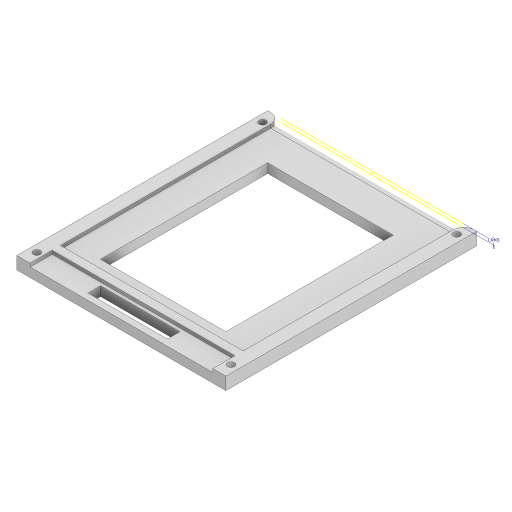
# Autodesk Inventor part: Scanner_Test_Bot
Saved by Autodesk Inventor 2023 (Build 270158000, 158)
## iProperties
Created: 2022-09-22
Part Number: Scanner_Test_Bot
Material: Generic
Document SubType Name: Modeling
Designer: Vking
Density: 1 g/cm^3
Appearance: Default
Author: Vking
Autodesk Inventor part; units mm, degrees
ref_plane "YZ Plane" through (0, 0, 0) normal (1, 0, 0) x (0, 1, 0)
ref_plane "XZ Plane" through (0, 0, 0) normal (0, 1, 0) x (-1, 0, 0)
ref_plane "XY Plane" through (0, 0, 0) normal (0, 0, 1) x (1, 0, 0)
sketch "Sketch1" plane through (0, 0, 0) normal (0, 0, 1) x (1, 0, 0)
  line L0 (-31.75, 5.08) -> (31.75, 5.08)
  line L1 (31.75, 5.08) -> (31.75, -5.08)
  line L2 (31.75, -5.08) -> (-31.75, -5.08)
  line L3 (-31.75, -5.08) -> (-31.75, 5.08)
  point P0 (0, 0)
  dimension "d0" = 63.5
  dimension "d3" = 31.75
  dimension "d4" = 10.16
  dimension "d17" = 5.08
  constraints: 8 end point, 2 parallel, 1 horizontal, 1 perpendicular
  measures "d0" distance of L0.start L0.end
  measures "d3" distance from line of L3 point (0, 0)
  measures "d4" distance of L0.end L1.end
  measures "d17" distance from line of point (0, 0) L2
extrude "Extrusion1" add sketch "Sketch1" along normal blind 76.2
sketch "Sketch3" plane through (0, 0, 76.2) normal (0, 0, 1) x (1, 0, 0)
  line L0 (-27.75, 0.3875) -> (27.75, 0.3875)
  line L1 (27.75, 0.3875) -> (27.75, -0.3745)
  line L2 (27.75, -0.3745) -> (-27.75, -0.3745)
  line L3 (-27.75, -0.3745) -> (-27.75, 0.3875)
  line L4 (-31.75, 5.08) -> (-31.75, -5.08) projected
  point P0 (0, 0)
  point P1 (-27.75, 0.0065)
  dimension "d6" = 0.762
  dimension "d7" = 55.5
  dimension "d8" = 4
  constraints: 8 end point, 2 parallel, 1 horizontal, 1 midpoint, 1 perpendicular
  measures "d6" distance between parallel lines of L2 L0
  measures "d7" distance of L0.start L0.end
  measures "d8" distance from line of L4 point (-27.75, 0.006)
extrude "Extrusion2" cut sketch "Sketch3" against normal blind 85.1
sketch "Sketch8" plane through (0, 0, 76.2) normal (0, 0, 1) x (1, 0, 0)
  line L0 (27.75, 0.3875) -> (27.75, -0.3745) projected
  line L1 (27.75, -0.3745) -> (-27.75, -0.3745) projected
  line L2 (-27.75, -0.3745) -> (-27.75, 0.3875) projected
  line L3 (-27.75, 0.3875) -> (27.75, 0.3875) projected
  line L4 (-31.75, -5.08) -> (31.75, -5.08) projected
  line L5 (31.75, -5.08) -> (31.75, 5.08) projected
  line L6 (31.75, 5.08) -> (-31.75, 5.08) projected
  line L7 (-31.75, 5.08) -> (-31.75, -5.08) projected
  line L8 (-31.75, 5.08) -> (31.75, 5.08)
  line L9 (31.75, 5.08) -> (31.75, 0.3875)
  line L10 (31.75, 0.3875) -> (-31.75, 0.3875)
  line L11 (-31.75, 0.3875) -> (-31.75, 5.08)
  point P0 (0, 0)
  point P1 (-31.75, 0.3875)
  dimension "d30" = 0
  constraints: 8 end point, 2 parallel, 1 horizontal, 1 perpendicular, 1 point on line
  measures "d30" distance between parallel lines of L3 L10
extrude "Extrusion6" cut sketch "Sketch8" against normal blind 76.2 contours L3 L10 L7 L6 L5
sketch "Sketch9" plane through (0, 0, 76.2) normal (0, 0, 1) x (1, 0, 0)
  line L0 (-31.75, 0.3875) -> (-31.75, -5.08) projected
  line L1 (31.75, -5.08) -> (31.75, 0.3875) projected
  line L2 (-31.75, -5.08) -> (31.75, -5.08)
  line L3 (31.75, -5.08) -> (31.75, -3.175)
  line L4 (31.75, -3.175) -> (-31.75, -3.175)
  line L5 (-31.75, -3.175) -> (-31.75, -5.08)
  point P0 (0, 0)
  dimension "d33" = 1.905
  constraints: 8 end point, 2 parallel, 1 horizontal, 1 perpendicular, 1 point on line
  measures "d33" distance between parallel lines of L2 L4
extrude "Extrusion7" cut sketch "Sketch9" against normal blind 76.2
sketch "Sketch10" plane through (-27.75, -0.3745, 76.2) normal (0, 1, 0) x (1, 0, 0)
  line L0 (59.5, 76.2) -> (-4, 76.2) projected
  line L1 (-4, 76.2) -> (59.5, 76.2)
  line L2 (59.5, 76.2) -> (59.5, 0)
  line L3 (59.5, 0) -> (-4, 0)
  line L4 (-4, 0) -> (-4, 76.2)
  line L5 (8.7, 12.7) -> (46.8, 12.7)
  line L6 (46.8, 12.7) -> (46.8, 63.5)
  line L7 (46.8, 63.5) -> (8.7, 63.5)
  line L8 (8.7, 63.5) -> (8.7, 12.7)
  dimension "d46" = 12.7
  constraints: 16 end point, 4 parallel, 2 perpendicular, 1 horizontal, 3 other
  measures "d46" distance between parallel lines of L3 L5
extrude "Extrusion8" cut sketch "Sketch10" against normal blind 25.4 contours L8 L7 L6 L5
fillet "Fillet3" radius 3.175 3 edges at (0, -0.3745, 0) (-27.75, 0.0065, 0) (27.75, 0.0065, 0)
sketch "Sketch11" plane through (-27.75, -0.3745, 76.2) normal (0, 1, 0) x (1, 0, 0)
  line L0 (15.6845, 1.905) -> (39.8145, 1.905)
  line L1 (39.8145, 1.905) -> (39.8145, 5.715)
  line L2 (39.8145, 5.715) -> (15.6845, 5.715)
  line L3 (15.6845, 5.715) -> (15.6845, 1.905)
  line L4 (55.5, 0) -> (0, 0) projected
  line L5 (0, 0) -> (0, 73.025) projected
  line L6 (-4, 0) -> (-4, 76.2) projected
  point P0 (27.75, 76.2)
  dimension "d47" = 1.905
  dimension "d48" = 3.81
  dimension "d51" = 24.13
  dimension "d52" = 15.6845
  dimension "d67" = 19.6845
  constraints: 8 end point, 2 parallel, 1 horizontal, 1 perpendicular
  measures "d47" distance between parallel lines of L4 L0
  measures "d48" distance between parallel lines of L0 L2
  measures "d51" distance of L1.end L2.end
  measures "d52" distance between parallel lines of L5 L3
  measures "d67" distance between parallel lines of L6 L3
extrude "Extrusion9" cut sketch "Sketch11" against normal blind 25.4
sketch "Sketch13" plane through (-31.75, -3.175, 76.2) normal (0, -1, 0) x (1, 0, 0)
  circle A0 centre (61.25, -3.81) radius 1.05
  line L0 (63.5, 0) -> (59, 0)
  circle A1 centre (2.25, -3.81) radius 1.05
  line L1 (4.5, 0) -> (0, 0)
  circle A2 centre (61.25, -72.39) radius 1.05
  line L2 (59, -76.2) -> (63.5, -76.2)
  line L3 (59, 0) -> (59, -76.2)
  circle A3 centre (2.25, -72.39) radius 1.05
  line L4 (0, 0) -> (0, -76.2)
  line L5 (0, -76.2) -> (4.5, -76.2)
  line L6 (50.8, -12.7) -> (50.8, -63.5)
  line L7 (50.8, -63.5) -> (12.7, -63.5)
  line L8 (12.7, -63.5) -> (12.7, -12.7)
  line L9 (12.7, -12.7) -> (50.8, -12.7)
  line L10 (63.5, 0) -> (0, 0)
  line L11 (0, 0) -> (0, -76.2)
  line L12 (63.5, -76.2) -> (0, -76.2)
  line L13 (63.5, 0) -> (63.5, -76.2)
  point P0 (31.75, -76.2)
  point P1 (31.75, -76.2)
  dimension "d53" = 2.1
  dimension "d54" = 3.81
  dimension "d55" = 2.25
  dimension "d56" = 2.25
  dimension "d57" = 2.1
  dimension "d58" = 3.81
  dimension "d59" = 2.1
  dimension "d60" = 2.1
  dimension "d61" = 3.81
  dimension "d62" = 3.81
  dimension "d63" = 2.25
  dimension "d64" = 2.25
  constraints: 28 end point, 4 centre point, 1 coincident
  measures "d53" diameter of A2
  measures "d54" distance from line of L2 A2.centre
  measures "d55" distance from line of A2.centre L3
  measures "d56" distance from line of L4 A3.centre
  measures "d57" diameter of A3
  measures "d58" distance from line of L5 A3.centre
  measures "d59" diameter of A1
  measures "d60" diameter of A0
  measures "d61" distance from line of A1.centre L1
  measures "d62" distance from line of A0.centre L0
  measures "d63" distance from line of L3 A0.centre
  measures "d64" distance from line of L4 A1.centre
extrude "Extrusion10" cut sketch "Sketch13" against normal blind 25.4 contours A0 | A1 | A2 | A3
sketch "Sketch14" plane through (-31.75, 0.3875, 76.2) normal (0, 1, 0) x (1, 0, 0)
  circle A0 centre (2.25, 3.81) radius 1.05 projected
  circle A1 centre (2.25, 72.39) radius 1.05 projected
  arc A2 (4, 73.025) -> (0.825, 76.2) centre (0.825, 73.025) ccw projected
  line L0 (0, 76.2) -> (0.825, 76.2) projected
  line L1 (0, 0) -> (0, 76.2) projected
  line L2 (4, 0) -> (0, 0) projected
  line L3 (4, 0) -> (4, 73.025) projected
  circle A3 centre (61.25, 3.81) radius 1.05 projected
  circle A4 centre (61.25, 72.39) radius 1.05 projected
  arc A5 (62.675, 76.2) -> (59.5, 73.025) centre (62.675, 73.025) ccw projected
  line L4 (59.5, 0) -> (59.5, 73.025) projected
  line L5 (63.5, 0) -> (59.5, 0) projected
  line L6 (63.5, 76.2) -> (63.5, 0) projected
  line L7 (62.675, 76.2) -> (63.5, 76.2) projected
  point P0 (31.75, 76.2)
extrude "Extrusion11" add sketch "Sketch14" along normal blind 0.5
sketch "Sketch15" plane through (-27.75, -0.3745, 76.2) normal (0, 1, 0) x (1, 0, 0)
  line L0 (0, 0) -> (0, 73.025) projected
  line L1 (0, 6.715) -> (55.7227, 6.715)
  line L2 (55.7227, 6.715) -> (55.7227, 9.255)
  line L3 (55.7227, 9.255) -> (0, 9.255)
  line L4 (0, 9.255) -> (0, 6.715)
  line L5 (15.6845, 5.715) -> (39.8145, 5.715) projected
  point P0 (27.75, 76.2)
  point P1 (0, 9.255)
  dimension "d72" = 2.54
  dimension "d77" = 1
  constraints: 8 end point, 2 parallel, 1 horizontal, 1 perpendicular, 1 point on line
  measures "d72" distance between parallel lines of L1 L3
  measures "d77" distance between parallel lines of L5 L1
extrude "Extrusion12" add sketch "Sketch15" along normal blind 1.3
sketch "Sketch16" plane through (0, 0, 76.2) normal (0, 0, 1) x (1, 0, 0)
  line L0 (31.75, -3.175) -> (31.75, 0.8875) projected
  line L1 (-36.1102, 11.8694) -> (32.0392, 11.8694)
  line L2 (32.0392, 11.8694) -> (32.0392, 0.6335)
  line L3 (32.0392, 0.6335) -> (-36.1102, 0.6335)
  line L4 (-36.1102, 0.6335) -> (-36.1102, 11.8694)
  line L5 (-31.75, 0.8875) -> (-27.75, 0.8875) projected
  point P0 (0, 0)
  dimension "d79" = 0.254
  constraints: 8 end point, 2 parallel, 1 horizontal, 1 perpendicular
  measures "d79" distance between parallel lines of L3 L5
extrude "Extrusion13" cut sketch "Sketch16" against normal blind 254
sketch "Sketch18" plane through (0, 0, 0) normal (0, 0, -1) x (-1, 0, 0)
  line L0 (27.7501, -0.3745) -> (-27.7501, -0.3745) projected
  line L1 (27.75, 0.6335) -> (-27.75, 0.6335) projected
  point P0 (0, 0)
  dimension "d78" = 1.008
  measures "d78" distance between parallel lines of L0 L1
body "Solid1"
